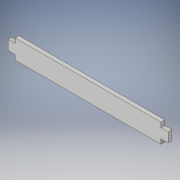
# Autodesk Inventor part: Jonction
Saved by Autodesk Inventor 2019.4 (Build 234330000, 330)
## iProperties
Created: 2019-12-15
Part Number: Jonction
Material: Generic
Document SubType Name: Modeling
Designer: fabfarm
Density: 1 g/cm^3
Appearance: Default
Author: fabfarm
Autodesk Inventor part; units mm, degrees
ref_plane "YZ Plane" through (0, 0, 0) normal (1, 0, 0) x (0, 1, 0)
ref_plane "XZ Plane" through (0, 0, 0) normal (0, 1, 0) x (-1, 0, 0)
ref_plane "XY Plane" through (0, 0, 0) normal (0, 0, 1) x (1, 0, 0)
sketch "Sketch1" plane through (0, 0, 0) normal (0, 0, 1) x (1, 0, 0)
  line L0 (0, 0) -> (759, 0)
  line L1 (759, 100) -> (0, 100)
  line L2 (0, 25) -> (-37.1, 25)
  line L3 (-37.1, 25) -> (-37.1, 75)
  line L4 (-37.1, 75) -> (0, 75)
  line L5 (759, 25) -> (796.1, 25)
  line L6 (796.1, 25) -> (796.1, 75)
  line L7 (796.1, 75) -> (759, 75)
  line L8 (0, 100) -> (0, 75)
  line L9 (0, 25) -> (0, 0)
  line L10 (759, 0) -> (759, 25)
  line L11 (759, 75) -> (759, 100)
  dimension "d0" = 100
  dimension "d1" = 759
  dimension "d2" = 25
  dimension "d3" = 25
  dimension "d5" = 37.1
  constraints: 24 end point, 7 parallel, 4 perpendicular, 3 collinear, 3 horizontal, 2 point on line
  measures "d0" distance of L1.end L0.start
  measures "d1" distance of L0.start L0.end
  measures "d2" distance between parallel lines of L1 L4
  measures "d3" distance between parallel lines of L0 L2
  measures "d5" distance between parallel lines of L3 L8
extrude "Extrusion1" add sketch "Sketch1" along normal blind 20.18
body "Solid1"
